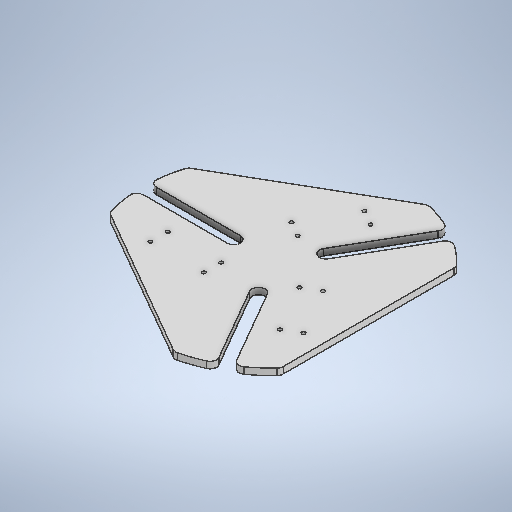
# Autodesk Inventor part: RT_FRM_SK_002_TopPlate
Saved by Autodesk Inventor 2025.3 (Build 293356000, 356)
## iProperties
Created: 2026-04-28
Part Number: RT_FRM_SK_002_TopPlate
Material: Generic
Document SubType Name: Modeling
Designer: louis
Density: 1 g/cm^3
Appearance: Default
Author: louis
Autodesk Inventor part; units mm, degrees
ref_plane "YZ Plane" through (0, 0, 0) normal (1, 0, 0) x (0, 1, 0)
ref_plane "XZ Plane" through (0, 0, 0) normal (0, 1, 0) x (-1, 0, 0)
ref_plane "XY Plane" through (0, 0, 0) normal (0, 0, 1) x (1, 0, 0)
sketch "Sketch1" plane through (0, 0, 0) normal (0, 1, 0) x (-1, 0, 0)
  line L0 (25, -2.5) -> (135, -2.5)
  line L1 (135, 0) -> (25, 0) construction
  line L2 (0, 0) -> (25, 0) construction
  circle A0 centre (0, 0) radius 200
  line L3 (50, 0) -> (103.8137, 0) construction
  line L4 (130, 26.5) -> (30, 26.5)
  line L5 (30, 26.5) -> (30, 76.5)
  line L6 (30, 76.5) -> (130, 76.5)
  line L7 (130, 76.5) -> (130, 26.5)
  line L8 (80, 26.5) -> (80, 0) construction
  line L9 (80, 76.5) -> (80, 26.5) construction
  line L10 (121, 40.5) -> (80, 40.5) construction
  line L11 (121, 40.5) -> (121, 67) construction
  line L12 (199.7498, -10) -> (50, -10)
  line L13 (50, -10) -> (50, 10)
  line L14 (50, 10) -> (199.7498, 10)
  line L15 (199.7498, 10) -> (199.7498, -10)
  line L16 (-33.6603, 38.3013) -> (-108.5352, 167.9884)
  line L17 (-91.2147, 177.9884) -> (-16.3397, 48.3013)
  line L18 (-16.3397, -48.3013) -> (-91.2147, -177.9884)
  line L19 (-108.5352, -167.9884) -> (-33.6603, -38.3013)
  line L20 (190.7878, -60) -> (-43.4324, -195.2271)
  line L21 (-43.4324, 195.2271) -> (190.7878, 60)
  line L22 (-147.3554, -135.2271) -> (-147.3554, 135.2271)
  point P0 (39, 40.5)
  point P1 (39, 67)
  dimension "d0" = 110
  dimension "d2" = 2.5
  dimension "d4" = 80
  dimension "d9" = 400
  dimension "d11" = 29
  dimension "d12" = 50
  dimension "d13" = 100
  dimension "d14" = 26.5
  dimension "d15" = 82
  dimension "d26" = 20
  dimension "d27" = 30
  dimension "d33" = 9.5
  dimension "d37" = 360
  dimension "d40" = 50
  dimension "d41" = 50
  dimension "d44" = 360
  constraints: 46 end point, 4 horizontal, 4 parallel, 4 point on circle, 3 midpoint, 3 perpendicular, 2 point on line, 2 symmetric about line, 2 vertical, 1 centre point, 1 coincident, 1 collinear, 29 other
  measures "d0" distance of L0.end L0.start
  measures "d2" distance between parallel lines of L0 L1
  measures "d4" distance of L2.start L8.end
  measures "d9" diameter of A0
  measures "d11" distance from line of L0 L4.start
  measures "d12" distance of L6.end L4.start
  measures "d13" distance of L4.start L4.end
  measures "d14" distance of L11.end L10.start
  measures "d15" distance of L10.start point (39, 40.5)
  measures "d26" distance between parallel lines of L14 L12
  measures "d27" distance between parallel lines of L8 L13
  measures "d33" distance from line of L6 L11.end
  measures "d40" distance from line of L12 L20.start
  measures "d41" distance from line of L18 L20.end
extrude "Extrusion1" add sketch "Sketch1" against normal blind 10 contours A0 L15 | L14 L13 L12 A0 L20 L22 L21 | L15 L12 L13 L14 | L4 L5 L6 L7
hole "Hole1" at (-121, 0, 40.5) at (-39, 0, 40.5) at (-121, 0, 67) at (-39, 0, 67) direction (0, -1, 0) diameter 5.5 end through all clearance for "Socket Head Cap Screw" size "M5" standard "Ansi Metric M Profile"
extrude "Extrusion2" cut sketch "Sketch1" against normal blind 10 contours A0 L15 | L15 L12 L13 L14
pattern_circular "Circular Pattern1" count 3 over 360 about axis through (0, -10, 0) along (0, 1, 0) of "Hole1", "Extrusion2"
fillet "Fillet1" radius 10 18 edges at (91.2147, -5, 177.9884) (16.3397, -5, 48.3013) (33.6603, -5, 38.3013) (108.5352, -5, 167.9884) (91.2147, -5, -177.9884) (16.3397, -5, -48.3013) (33.6603, -5, -38.3013) (108.5352, -5, -167.9884) (-199.7498, -5, 10) (-50, -5, 10) (-50, -5, -10) (-199.7498, -5, -10) (-190.7878, -5, 60) (43.4324, -5, 195.2271) (147.3554, -5, 135.2271) (147.3554, -5, -135.2271) (43.4324, -5, -195.2271) (-190.7878, -5, -60)
body "Solid1"
